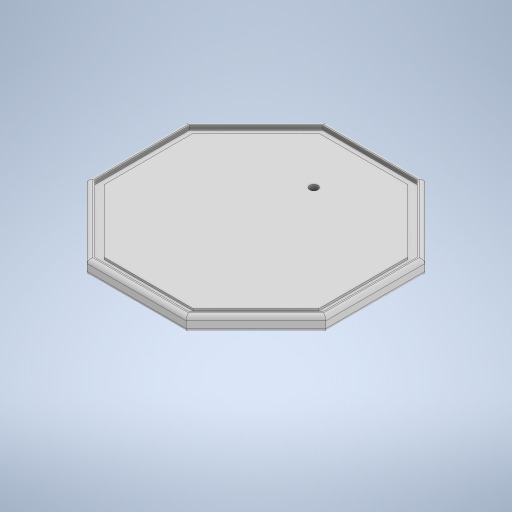
# Autodesk Inventor part: OV-PAM_top_2
Saved by Autodesk Inventor 2024 (Build 280153000, 153)
## iProperties
Created: 2023-06-16
Part Number: OV-PAM_top_2
Material: 일반
Document SubType Name: Modeling
Designer: jsw
Density: 1 g/cm^3
Appearance: 기본값
Author: jsw
Autodesk Inventor part; units mm, degrees
ref_plane "YZ Plane" through (0, 0, 0) normal (1, 0, 0) x (0, 1, 0)
ref_plane "XZ Plane" through (0, 0, 0) normal (0, 1, 0) x (-1, 0, 0)
ref_plane "XY Plane" through (0, 0, 0) normal (0, 0, 1) x (1, 0, 0)
sketch "스케치3" plane through (0, 0, 0) normal (0, 1, 0) x (-1, 0, 0)
  line L0 (35.7919, -14.8255) -> (14.8255, -35.7919)
  line L1 (14.8255, -35.7919) -> (-14.8255, -35.7919)
  line L2 (-14.8255, -35.7919) -> (-35.7919, -14.8255)
  line L3 (-35.7919, -14.8255) -> (-35.7919, 14.8255)
  line L4 (-35.7919, 14.8255) -> (-14.8255, 35.7919)
  line L5 (-14.8255, 35.7919) -> (14.8255, 35.7919)
  line L6 (14.8255, 35.7919) -> (35.7919, 14.8255)
  line L7 (35.7919, 14.8255) -> (35.7919, -14.8255)
  line L8 (32.5919, -13.5) -> (13.5, -32.5919)
  line L9 (13.5, -32.5919) -> (-13.5, -32.5919)
  line L10 (-13.5, -32.5919) -> (-32.5919, -13.5)
  line L11 (-32.5919, -13.5) -> (-32.5919, 13.5)
  line L12 (-32.5919, 13.5) -> (-13.5, 32.5919)
  line L13 (-13.5, 32.5919) -> (13.5, 32.5919)
  line L14 (13.5, 32.5919) -> (32.5919, 13.5)
  line L15 (32.5919, 13.5) -> (32.5919, -13.5)
  point P0 (0, 0)
  point P1 (0, 0)
  point P2 (0, 0)
  point P3 (0, 0)
  dimension "d43" = 27
  dimension "d44" = 3.2
  constraints: 32 end point, 3 coincident, 2 horizontal, 34 other
  measures "d43" distance of L8.end L9.end
  measures "d44" distance between parallel lines of L7 L15
extrude "돌출2" add sketch "스케치3" along normal blind 4.4 contours L0 L1 L2 L3 L4 L5 L6 L7 | L8 L9 L10 L11 L12 L13 L14 L15
sketch "스케치4" plane through (0, 4.4, 0) normal (0, 1, 0) x (1, 0, 0)
  line L0 (13.5, -32.5919) -> (-13.5, -32.5919)
  line L1 (-13.5, -32.5919) -> (-32.5919, -13.5)
  line L2 (-32.5919, -13.5) -> (-32.5919, 13.5)
  line L3 (-32.5919, 13.5) -> (-13.5, 32.5919)
  line L4 (-13.5, 32.5919) -> (13.5, 32.5919)
  line L5 (13.5, 32.5919) -> (32.5919, 13.5)
  line L6 (32.5919, 13.5) -> (32.5919, -13.5)
  line L7 (32.5919, -13.5) -> (13.5, -32.5919)
  line L8 (-14.1627, 34.1919) -> (14.1627, 34.1919)
  line L9 (14.1627, 34.1919) -> (34.1919, 14.1627)
  line L10 (34.1919, 14.1627) -> (34.1919, -14.1627)
  line L11 (34.1919, -14.1627) -> (14.1627, -34.1919)
  line L12 (14.1627, -34.1919) -> (-14.1627, -34.1919)
  line L13 (-14.1627, -34.1919) -> (-34.1919, -14.1627)
  line L14 (-34.1919, -14.1627) -> (-34.1919, 14.1627)
  line L15 (-34.1919, 14.1627) -> (-14.1627, 34.1919)
  line L16 (-13.3343, 32.1919) -> (13.3343, 32.1919)
  line L17 (13.3343, 32.1919) -> (32.1919, 13.3343)
  line L18 (32.1919, 13.3343) -> (32.1919, -13.3343)
  line L19 (32.1919, -13.3343) -> (13.3343, -32.1919)
  line L20 (13.3343, -32.1919) -> (-13.3343, -32.1919)
  line L21 (-13.3343, -32.1919) -> (-32.1919, -13.3343)
  line L22 (-32.1919, -13.3343) -> (-32.1919, 13.3343)
  line L23 (-32.1919, 13.3343) -> (-13.3343, 32.1919)
  line L24 (-35.7919, 14.8255) -> (-35.7919, -14.8255) projected
  point P0 (0, 0)
  point P1 (0, 0)
  point P2 (0, 0)
  point P3 (0, 0)
  dimension "d7" = 27
  dimension "d60" = 1.6
  dimension "d61" = 2
  constraints: 48 end point, 3 coincident, 3 horizontal, 51 other
  measures "d7" distance of L1.end L2.end
  measures "d60" distance between parallel lines of L14 L24
  measures "d61" distance between parallel lines of L14 L22
extrude "돌출3" cut sketch "스케치4" against normal blind 1.2 contours L0 L1 L2 L3 L4 L5 L6 L7 | L8 L9 L10 L11 L12 L13 L14 L15 | L16 L17 L18 L19 L20 L21 L22 L23
sketch "스케치5" plane through (0, 0, 0) normal (0, -1, 0) x (1, 0, 0)
  line L0 (10, 2.5) -> (20, 2.5)
  line L1 (20, 2.5) -> (20, -2.5)
  line L2 (20, -2.5) -> (10, -2.5)
  line L3 (10, -2.5) -> (10, 2.5)
  line L4 (10, 2.5) -> (20, -2.5) construction
  line L5 (20, 2.5) -> (10, -2.5) construction
  line L6 (-20, 2.5) -> (-10, 2.5)
  line L7 (-10, 2.5) -> (-10, -2.5)
  line L8 (-10, -2.5) -> (-20, -2.5)
  line L9 (-20, -2.5) -> (-20, 2.5)
  line L10 (-20, 2.5) -> (-10, -2.5) construction
  line L11 (-10, 2.5) -> (-20, -2.5) construction
  point P0 (0, 0)
  point P1 (15, 0)
  point P2 (-15, 0)
  dimension "d11" = 10
  dimension "d12" = 5
  dimension "d13" = 10
  dimension "d16" = 30
  constraints: 24 end point, 2 horizontal, 2 midpoint, 2 parallel, 1 collinear, 1 horizontal alignment, 1 perpendicular, 10 other
  measures "d11" distance of L1.end L2.end
  measures "d12" distance of L0.end L1.end
  measures "d13" distance from line of L3 point (0, 0)
  measures "d16" distance of L0.start L6.start
extrude "돌출4" add sketch "스케치5" along normal blind 10
sketch "스케치6" plane through (-10, 0, -2.5) normal (0, 0, -1) x (-1, 0, 0)
  circle A0 centre (5, -10) radius 5
  circle A1 centre (-25, -10) radius 5
  line L0 (-20, -10) -> (-30, -10) projected
  line L1 (10, -10) -> (0, -10) projected
  point P0 (-10, 0)
  dimension "d23" = 10
  dimension "d24" = 10
  constraints: 2 centre point, 2 coincident, 2 midpoint
  measures "d23" diameter of A0
  measures "d24" diameter of A1
extrude "돌출5" add sketch "스케치6" against normal blind 5
sketch "스케치7" plane through (-10, 0, -2.5) normal (0, 0, -1) x (-1, 0, 0)
  circle A0 centre (5, -10) radius 1.25
  line L0 (10, 0) -> (10, -10) projected
  line L1 (0, 0) -> (10, 0) projected
  line L2 (4.7788, 0) -> (0, 0)
  circle A1 centre (-25, -10) radius 1.25
  point P0 (-10, 0)
  dimension "d27" = 2.5
  dimension "d28" = 5
  dimension "d31" = 30
  constraints: 2 centre point, 2 end point, 1 horizontal, 1 horizontal alignment, 1 point on line, 2 other
  measures "d27" diameter of A0
  measures "d28" distance from line of L0 A0.centre
  measures "d31" distance of A0.centre A1.centre
extrude "돌출6" cut sketch "스케치7" against normal blind 5
sketch "스케치8" plane through (0, 0, 0) normal (0, -1, 0) x (1, 0, 0)
  circle A0 centre (0, -17.3205) radius 1.25
  line L0 (-10, 2.5) -> (-10, -2.5) projected
  point P0 (0, 0)
  point P1 (-10, 0)
  dimension "d38" = 2.5
  dimension "d39" = 17.3205
  constraints: 1 centre point, 1 midpoint, 1 vertical alignment
  measures "d38" diameter of A0
  measures "d39" vertical distance of A0.centre point (-10, 0)
sketch "스케치9" plane through (0, 3.2, 0) normal (0, 1, 0) x (1, 0, 0)
  line L0 (-13.3343, 32.1919) -> (13.3343, 32.1919)
  line L1 (13.3343, 32.1919) -> (32.1919, 13.3343)
  line L2 (32.1919, 13.3343) -> (32.1919, -13.3343)
  line L3 (32.1919, -13.3343) -> (13.3343, -32.1919)
  line L4 (13.3343, -32.1919) -> (-13.3343, -32.1919)
  line L5 (-13.3343, -32.1919) -> (-32.1919, -13.3343)
  line L6 (-32.1919, -13.3343) -> (-32.1919, 13.3343)
  line L7 (-32.1919, 13.3343) -> (-13.3343, 32.1919)
  line L8 (-14.1627, 34.1919) -> (14.1627, 34.1919) projected
  line L9 (-12.0917, 29.1919) -> (12.0917, 29.1919)
  line L10 (12.0917, 29.1919) -> (29.1919, 12.0917)
  line L11 (29.1919, 12.0917) -> (29.1919, -12.0917)
  line L12 (29.1919, -12.0917) -> (12.0917, -29.1919)
  line L13 (12.0917, -29.1919) -> (-12.0917, -29.1919)
  line L14 (-12.0917, -29.1919) -> (-29.1919, -12.0917)
  line L15 (-29.1919, -12.0917) -> (-29.1919, 12.0917)
  line L16 (-29.1919, 12.0917) -> (-12.0917, 29.1919)
  point P0 (0, 0)
  point P1 (0, 0)
  point P2 (0, 0)
  dimension "d46" = 2
  dimension "d47" = 3
  constraints: 32 end point, 2 coincident, 2 horizontal, 34 other
  measures "d46" distance between parallel lines of L0 L8
  measures "d47" distance between parallel lines of L0 L9
extrude "돌출8" add sketch "스케치9" along normal blind 0.6 contours L0 L1 L2 L3 L4 L5 L6 L7 | L9 L10 L11 L12 L13 L14 L15 L16
fillet "모깎기1" radius 1.2 16 edges at (-35.7919, 4.4, 0) (-25.3087, 4.4, 25.3087) (0, 4.4, 35.7919) (25.3087, 4.4, 25.3087) (35.7919, 4.4, 0) (25.3087, 4.4, -25.3087) (0, 4.4, -35.7919) (-25.3087, 4.4, -25.3087) (25.3087, 0, 25.3087) (0, 0, 35.7919) (-25.3087, 0, 25.3087) (-35.7919, 0, 0) (-25.3087, 0, -25.3087) (0, 0, -35.7919) (25.3087, 0, -25.3087) (35.7919, 0, 0)
sketch "스케치10" plane through (0, 0, 0) normal (0, -1, 0) x (1, 0, 0)
  line L0 (-20, 2.5) -> (-10, 2.5) projected
  line L1 (-10, -2.5) -> (-20, -2.5) projected
  line L2 (-20, 2.5) -> (-19, 2.5)
  line L3 (-19, 2.5) -> (-19, -2.5)
  line L4 (-19, -2.5) -> (-20, -2.5)
  line L5 (-20, -2.5) -> (-20, 2.5)
  line L6 (20, -2.5) -> (10, -2.5) projected
  line L7 (10, 2.5) -> (20, 2.5) projected
  line L8 (20, -2.5) -> (19, -2.5)
  line L9 (19, -2.5) -> (19, 2.5)
  line L10 (19, 2.5) -> (20, 2.5)
  line L11 (20, 2.5) -> (20, -2.5)
  point P0 (0, 0)
  dimension "d54" = 1
  dimension "d55" = 1
  constraints: 16 end point, 4 parallel, 2 horizontal, 2 perpendicular, 2 point on line
  measures "d54" distance of L1.end L3.end
  measures "d55" distance of L9.end L10.end
extrude "돌출9" cut sketch "스케치10" along normal blind 15
extrude "돌출10" cut sketch "스케치8" against normal blind 5
equation "\"d55\" = d54"
